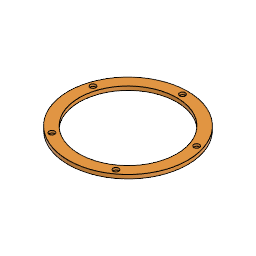
Frame-cap (Autodesk Fusion 360 design; units mm, degrees)
part number: 2026-05-19-16-44-30-295
Autodesk Fusion 360 part; units mm, degrees
sketch "Sketch1" plane through (0, 0, 0) normal (0, 0, 1) x (1, 0, 0)
  circle A0 centre (0, 0) radius 44
  circle A1 centre (0, 0) radius 54
  line L0 (0, 0) -> (0, 49.2393) construction
  circle A2 centre (0, 49.2393) radius 2.5
  circle A3 centre (-46.8293, 15.2158) radius 2.5
  circle A4 centre (-28.9421, -39.8354) radius 2.5
  circle A5 centre (28.9421, -39.8354) radius 2.5
  circle A6 centre (46.8293, 15.2158) radius 2.5
  dimension "d1" = 88
  dimension "d2" = 108
  dimension "d3" = 49.2393
  dimension "d4" = 5
  dimension "d6" = 360
  constraint coincident A0.centre A1.centre
  constraint concentric A0 A1
  constraint vertical L0
  constraint coincident L0.end A2.centre
  measures "d1" diameter of A0
  measures "d2" diameter of A1
  measures "d3" distance of A0.centre L0.end
  measures "d4" diameter of A2
extrude "Extrude1" add sketch "Sketch1" along normal blind 1.5 contours A2 | A3 | A4 | A5 | A6 makes body 1 at (49.3262, 15.0912, 1) makes body 2 at (2.4969, 49.1147, 1) makes body 3 at (31.439, -39.96, 1) makes body 4 at (-44.3324, 15.0912, 1) makes body 5 at (-26.4452, -39.96, 1)
extrude "Extrude2" add sketch "Sketch1" along normal blind 3.5 bodies 1 2 3 4 5
